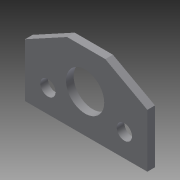
# Autodesk Inventor part: 2.3 Tutorial
Saved by Autodesk Inventor 2015 (Build 190159000, 159)
## iProperties
Created: 2015-09-02
Part Number: 2.3 Tutorial
Material: Generic
Document SubType Name: Modeling
Designer: Brandon
Density: 1 g/cm^3
Appearance: Default
Author: Brandon
Autodesk Inventor part; units mm, degrees
ref_plane "YZ Plane" through (0, 0, 0) normal (1, 0, 0) x (0, 1, 0)
ref_plane "XZ Plane" through (0, 0, 0) normal (0, 1, 0) x (-1, 0, 0)
ref_plane "XY Plane" through (0, 0, 0) normal (0, 0, 1) x (1, 0, 0)
sketch "Sketch1" plane through (0, 0, 0) normal (0, 0, 1) x (1, 0, 0)
  point P0 (0, 0)
sketch "Sketch2" plane through (0, 0, 0) normal (0, 0, 1) x (1, 0, 0)
  line L0 (0, 0) -> (101.6, 0)
  line L1 (101.6, 0) -> (101.6, 44.45)
  line L2 (0, 0) -> (0, 44.45)
  line L3 (34.925, 63.5) -> (66.675, 63.5)
  line L4 (66.675, 63.5) -> (101.6, 44.45)
  line L5 (34.925, 63.5) -> (0, 44.45)
  circle A0 centre (82.55, 19.05) radius 6.35
  circle A1 centre (19.05, 19.05) radius 6.35
  circle A2 centre (49.9058, 31.75) radius 15.875
  dimension "d1" = 44.45
  dimension "d2" = 44.45
  dimension "d6" = 31.75
  dimension "d7" = 63.5
  dimension "d9" = 19.05
  dimension "d10" = 19.05
  dimension "d12" = 19.05
  dimension "d13" = 12.7
  dimension "d14" = 19.05
  dimension "d15" = 12.7
  dimension "d16" = 31.75
  dimension "d17" = 31.75
  constraints: 12 end point, 3 centre point, 1 horizontal, 1 perpendicular, 1 vertical
  measures "d1" distance of L0.end L1.end
  measures "d2" distance of L0.start L2.end
  measures "d6" distance of L3.start L3.end
  measures "d7" vertical distance of L3.start L0.start
  measures "d9" horizontal distance of L1.end A0.centre
  measures "d10" horizontal distance of L0.end A0.centre
  measures "d12" horizontal distance of L0.start A1.centre
  measures "d13" diameter of A1
  measures "d14" horizontal distance of L2.end A1.centre
  measures "d15" diameter of A0
  measures "d16" diameter of A2
  measures "d17" vertical distance of L0.end A2.centre
sketch "Sketch3" plane through (0, 0, 0) normal (0, 0, 1) x (1, 0, 0)
  point P0 (0, 0)
extrude "Extrusion1" add sketch "Sketch2" along normal blind 6.35
body "Solid1"
